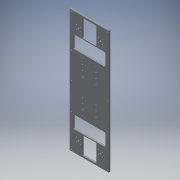
# Autodesk Inventor part: socle_ammovible
Saved by Autodesk Inventor 2017 (Build 210142000, 142)
## iProperties
Created: 2017-12-17
Part Number: socle_ammovible
Material: Generic
Document SubType Name: Modeling
Designer: franc
Density: 1 g/cm^3
Appearance: Default
Mass: 76.8943 g
Surface Area: 459.65 cm^2
Volume: 76.8943 cm^3
Author: franc
Autodesk Inventor part; units mm, degrees
ref_plane "YZ Plane" through (0, 0, 0) normal (1, 0, 0) x (0, 1, 0)
ref_plane "XZ Plane" through (0, 0, 0) normal (0, 1, 0) x (-1, 0, 0)
ref_plane "XY Plane" through (0, 0, 0) normal (0, 0, 1) x (1, 0, 0)
sketch "Esquisse1" plane through (0, 0, 0) normal (0, 1, 0) x (-1, 0, 0)
  line L0 (65.6569, 117.587) -> (-26.3431, 117.587)
  line L1 (-26.3431, 117.587) -> (-26.3431, -172.413)
  line L2 (-26.3431, -172.413) -> (65.6569, -172.413)
  line L3 (65.6569, -172.413) -> (65.6569, 117.587)
  line L4 (55.6569, 69.587) -> (-16.3431, 69.587)
  line L5 (-18.3431, 67.587) -> (-18.3431, 41.587)
  line L6 (-16.3431, 39.587) -> (55.6569, 39.587)
  line L7 (57.6569, 41.587) -> (57.6569, 67.587)
  arc A0 (-18.3431, 41.587) -> (-16.3431, 39.587) centre (-16.3431, 41.587) ccw
  arc A1 (55.6569, 39.587) -> (57.6569, 41.587) centre (55.6569, 41.587) ccw
  arc A2 (57.6569, 67.587) -> (55.6569, 69.587) centre (55.6569, 67.587) ccw
  arc A3 (-16.3431, 69.587) -> (-18.3431, 67.587) centre (-16.3431, 67.587) ccw
  line L8 (65.6569, -27.413) -> (-26.3431, -27.413) construction
  line L9 (55.6569, -124.413) -> (-16.3431, -124.413)
  line L10 (-18.3431, -122.413) -> (-18.3431, -96.413)
  line L11 (-16.3431, -94.413) -> (55.6569, -94.413)
  line L12 (57.6569, -96.413) -> (57.6569, -122.413)
  arc A4 (-16.3431, -94.413) -> (-18.3431, -96.413) centre (-16.3431, -96.413) ccw
  arc A5 (57.6569, -96.413) -> (55.6569, -94.413) centre (55.6569, -96.413) ccw
  arc A6 (55.6569, -124.413) -> (57.6569, -122.413) centre (55.6569, -122.413) ccw
  arc A7 (-18.3431, -122.413) -> (-16.3431, -124.413) centre (-16.3431, -122.413) ccw
  point P0 (0, 0)
  dimension "d0" = 290
  dimension "d1" = 92
  dimension "d7" = 30
  dimension "d8" = 8
  dimension "d9" = 8
  dimension "d10" = 2
  dimension "d15" = 48
  dimension "d23" = 145
  constraints: 26 end point, 16 point on circle, 12 symmetric about line, 8 centre point, 8 tangent, 4 parallel, 3 equal radius, 3 perpendicular, 2 horizontal, 2 midpoint, 4 other
  measures "d0" distance of L2.end L0.start
  measures "d1" distance of L0.start L0.end
  measures "d7" distance between parallel lines of L4 L6
  measures "d8" distance between parallel lines of L7 L3
  measures "d9" distance between parallel lines of L1 L5
  measures "d10" radius of A0
  measures "d15" distance between parallel lines of L0 L4
  measures "d23" distance between parallel lines of L8 L0
extrude "Extrusion1" add sketch "Esquisse1" along normal blind 4
sketch "Esquisse3" plane through (0, 4, 0) normal (0, 1, 0) x (1, 0, 0)
  circle A0 centre (-35.2599, -31.2495) radius 1.5875 projected
  circle A1 centre (-35.2599, -18.5495) radius 1.5875 projected
  circle A2 centre (-35.2599, -5.8495) radius 1.5875 projected
  arc A3 (-57.6569, 96.413) -> (-55.6569, 94.413) centre (-55.6569, 96.413) ccw projected
  line L0 (-57.6569, 96.413) -> (-57.6569, 122.413) projected
  arc A4 (-55.6569, 124.413) -> (-57.6569, 122.413) centre (-55.6569, 122.413) ccw projected
  line L1 (-55.6569, 124.413) -> (16.3431, 124.413) projected
  arc A5 (18.3431, 122.413) -> (16.3431, 124.413) centre (16.3431, 122.413) ccw projected
  line L2 (18.3431, 122.413) -> (18.3431, 96.413) projected
  arc A6 (16.3431, 94.413) -> (18.3431, 96.413) centre (16.3431, 96.413) ccw projected
  line L3 (16.3431, 94.413) -> (-55.6569, 94.413) projected
  arc A7 (16.3431, -69.587) -> (18.3431, -67.587) centre (16.3431, -67.587) ccw projected
  line L4 (16.3431, -69.587) -> (-55.6569, -69.587) projected
  arc A8 (-57.6569, -67.587) -> (-55.6569, -69.587) centre (-55.6569, -67.587) ccw projected
  line L5 (-57.6569, -67.587) -> (-57.6569, -41.587) projected
  arc A9 (-55.6569, -39.587) -> (-57.6569, -41.587) centre (-55.6569, -41.587) ccw projected
  line L6 (-55.6569, -39.587) -> (16.3431, -39.587) projected
  arc A10 (18.3431, -41.587) -> (16.3431, -39.587) centre (16.3431, -41.587) ccw projected
  line L7 (18.3431, -41.587) -> (18.3431, -67.587) projected
  line L8 (-65.6569, -117.587) -> (26.3431, -117.587) projected
  line L9 (26.3431, -117.587) -> (26.3431, 172.413) projected
  line L10 (26.3431, 172.413) -> (-65.6569, 172.413) projected
  line L11 (-65.6569, 172.413) -> (-65.6569, -117.587) projected
  circle A11 centre (-35.2599, 6.8505) radius 1.5875 projected
  circle A12 centre (-4.0179, -31.2495) radius 1.5875 projected
  circle A13 centre (-4.0179, -18.5495) radius 1.5875 projected
  circle A14 centre (-4.0179, -5.8495) radius 1.5875 projected
  circle A15 centre (-4.0179, 6.8505) radius 1.5875 projected
extrude "Extrusion3" cut sketch "Esquisse3" against normal through all contours A0 | A1 | A2 | A11 | A12 | A13 | A14 | A15
ref_plane "Plan médian largeur" through (-65.6569, 0, -27.413) normal (0, 0, 1) x (1, 0, 0)
sketch "Esquisse4" plane through (0, 4, 0) normal (0, 1, 0) x (1, 0, 0)
  line L0 (-34.6569, -71.587) -> (-4.6569, -71.587)
  line L1 (-2.6569, -73.587) -> (-2.6569, -111.587)
  line L2 (16.3431, -69.587) -> (-55.6569, -69.587) projected
  line L3 (-36.6569, -73.587) -> (-36.6569, -111.587)
  line L4 (-65.6569, 172.413) -> (-65.6569, -117.587) projected
  line L5 (-34.6569, -113.587) -> (-4.6569, -113.587)
  arc A0 (-36.6569, -111.587) -> (-34.6569, -113.587) centre (-34.6569, -111.587) ccw
  arc A1 (-4.6569, -113.587) -> (-2.6569, -111.587) centre (-4.6569, -111.587) ccw
  arc A2 (-2.6569, -73.587) -> (-4.6569, -71.587) centre (-4.6569, -73.587) ccw
  arc A3 (-34.6569, -71.587) -> (-36.6569, -73.587) centre (-34.6569, -73.587) ccw
  point P0 (0, 0)
  point P1 (-36.6569, -71.587)
  point P2 (-2.6569, -71.587)
  point P3 (-36.6569, -113.587)
  dimension "d24" = 34
  dimension "d25" = 42
  dimension "d29" = 2
  dimension "d52" = 2
  dimension "d53" = 29
  constraints: 8 end point, 8 point on circle, 8 tangent, 6 point on line, 4 centre point, 3 equal radius, 1 horizontal, 1 perpendicular, 1 vertical
  measures "d24" distance of point (-36.657, -71.587) point (-2.657, -71.587)
  measures "d25" distance of point (-36.657, -71.587) point (-36.657, -113.587)
  measures "d29" distance between parallel lines of L2 L0
  measures "d52" radius of A0
  measures "d53" distance between parallel lines of L4 L3
extrude "Extrusion4" cut sketch "Esquisse4" against normal through all
sketch "Esquisse6" plane through (0, 0, 0) normal (0, -1, 0) x (1, 0, 0)
  circle A0 centre (-61.6569, 113.587) radius 1.5
  circle A1 centre (22.3431, 113.587) radius 1.5
  circle A2 centre (22.3431, 35.587) radius 1.5
  circle A3 centre (-61.6569, 35.587) radius 1.5
  circle A4 centre (-61.6569, -27.413) radius 1.5
  circle A5 centre (22.3431, -27.413) radius 1.5
  line L0 (-65.6569, -172.413) -> (-65.6569, 117.587) projected
  line L1 (-65.6569, 117.587) -> (26.3431, 117.587) projected
  line L2 (26.3431, 117.587) -> (26.3431, -172.413) projected
  line L3 (16.3431, 39.587) -> (-55.6569, 39.587) projected
  point P0 (0, 0)
  dimension "d32" = 3
  dimension "d33" = 3
  dimension "d34" = 3
  dimension "d35" = 3
  dimension "d36" = 3
  dimension "d37" = 3
  dimension "d38" = 4
  dimension "d39" = 4
  dimension "d40" = 4
  dimension "d41" = 4
  dimension "d42" = 4
  dimension "d43" = 4
  dimension "d44" = 4
  dimension "d45" = 4
  dimension "d46" = 4
  dimension "d47" = 145
  dimension "d48" = 145
  dimension "d49" = 4
  constraints: 6 centre point
  measures "d32" diameter of A4
  measures "d33" diameter of A3
  measures "d34" diameter of A0
  measures "d35" diameter of A1
  measures "d36" diameter of A2
  measures "d37" diameter of A5
  measures "d38" distance from line of L0 A0.centre
  measures "d39" distance from line of L1 A0.centre
  measures "d40" distance from line of L2 A1.centre
  measures "d41" distance from line of L1 A1.centre
  measures "d42" distance from line of L2 A2.centre
  measures "d43" distance from line of L3 A2.centre
  measures "d44" distance from line of L0 A3.centre
  measures "d45" distance from line of L3 A3.centre
  measures "d46" distance from line of L0 A4.centre
  measures "d47" distance from line of L1 A4.centre
  measures "d48" distance from line of L1 A5.centre
  measures "d49" distance from line of L2 A5.centre
extrude "Extrusion5" cut sketch "Esquisse6" against normal through all
sketch "Esquisse7" plane through (0, 4, 0) normal (0, 1, 0) x (1, 0, 0)
  circle A0 centre (11.3431, -92.587) radius 1.9 projected
  circle A1 centre (11.3431, -82.587) radius 1.9 projected
  circle A2 centre (6.3431, -87.587) radius 4.25 projected
  circle A3 centre (-40.6569, -92.587) radius 1.9 projected
  circle A4 centre (1.3431, -92.587) radius 1.9 projected
  circle A5 centre (1.3431, -82.587) radius 1.9 projected
  circle A6 centre (11.3431, -92.587) radius 1.5
  circle A7 centre (1.3431, -92.587) radius 1.5
  circle A8 centre (6.3431, -87.587) radius 2.5
  circle A9 centre (1.3431, -82.587) radius 1.5
  circle A10 centre (11.3431, -82.587) radius 1.5
  circle A11 centre (-50.6569, -92.587) radius 1.5 projected
  circle A12 centre (-50.6569, -82.587) radius 1.5 projected
  circle A13 centre (-40.6569, -82.587) radius 1.5 projected
  circle A14 centre (-45.6569, -87.587) radius 2.75 projected
  circle A15 centre (-40.6569, -92.587) radius 1.5
  circle A16 centre (-50.6569, -92.587) radius 1.5
  circle A17 centre (-50.6569, -82.587) radius 1.5
  circle A18 centre (-40.6569, -82.587) radius 1.5
  circle A19 centre (-45.6569, -87.587) radius 2.5
  point P0 (0, 0)
  dimension "d55" = 3
  dimension "d56" = 3
  dimension "d57" = 5
  dimension "d58" = 3
  dimension "d59" = 3
  dimension "d60" = 3
  dimension "d61" = 3
  dimension "d62" = 3
  dimension "d63" = 3
  dimension "d64" = 5
  constraints: 10 centre point, 10 coincident
  measures "d55" diameter of A6
  measures "d56" diameter of A7
  measures "d57" diameter of A8
  measures "d58" diameter of A9
  measures "d59" diameter of A10
  measures "d60" diameter of A15
  measures "d61" diameter of A16
  measures "d62" diameter of A17
  measures "d63" diameter of A18
  measures "d64" diameter of A19
extrude "Extrusion6" cut sketch "Esquisse7" against normal through all contours A6 | A7 | A8 | A9 | A10 | A11 | A12 | A13 | A15 | A19
mirror "Symétrie1" about plane through (-65.6569, 0, -27.413) normal (0, 0, 1) of "Extrusion3", "Extrusion4", "Extrusion5", "Extrusion6"
equation "\"d23\" = 0.5 * d0"
